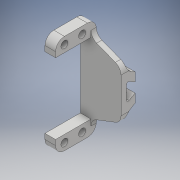
# Autodesk Inventor part: bigServoHolder2
Saved by Autodesk Inventor 2017 (Build 210142000, 142)
## iProperties
Created: 2017-01-16
Part Number: bigServoHolder2
Material: Generic
Document SubType Name: Modeling
Designer: Andi
Density: 1 g/cm^3
Appearance: Default
Author: Andi
Autodesk Inventor part; units mm, degrees
ref_plane "YZ Plane" through (0, 0, 0) normal (1, 0, 0) x (0, 1, 0)
ref_plane "XZ Plane" through (0, 0, 0) normal (0, 1, 0) x (-1, 0, 0)
ref_plane "XY Plane" through (0, 0, 0) normal (0, 0, 1) x (1, 0, 0)
sketch "Sketch1" plane through (0, 0, 0) normal (1, 0, 0) x (0, 1, 0)
  line L0 (0, 0) -> (0, 40)
  line L1 (0, 40) -> (-20, 40)
  line L2 (-20, 40) -> (-20, 43)
  line L3 (-15, 48) -> (-2, 48)
  line L4 (-2, -8) -> (-15, -8)
  line L5 (-20, -3) -> (-20, 0)
  line L6 (-20, 0) -> (0, 0)
  line L7 (0, 20) -> (3, 20)
  line L8 (3, 20) -> (3, 25.5)
  line L9 (3, 23.7768) -> (3, 20)
  line L10 (3, 20) -> (3, 16.2232)
  line L11 (3, 20) -> (7.9, 20)
  line L12 (7.9, 20) -> (7.9, 22.7)
  line L13 (7.9, 22.7) -> (7.9, 20)
  line L14 (7.9, 20) -> (7.9, 17.3)
  line L15 (7.9, 20) -> (10.6, 20) construction
  line L16 (4.4961, 24.6451) -> (7.9, 22.7)
  line L17 (7.9, 17.3) -> (4.4961, 15.3549)
  line L18 (7.9, 17.3) -> (7.9, 12.3)
  line L19 (7.9, 12.3) -> (5.5193, 10.9396)
  line L20 (7.9, 22.7) -> (7.9, 27.7)
  line L21 (7.9, 27.7) -> (5.5193, 29.0604)
  line L22 (3, 43) -> (3, 33.4016)
  line L23 (3, 30.5) -> (3, 25.5)
  line L24 (3, 14.5) -> (3, 9.5)
  line L25 (3, 6.5984) -> (3, -3)
  arc A0 (3, 33.4016) -> (5.5193, 29.0604) centre (8, 33.4016) ccw
  arc A1 (5.5193, 10.9396) -> (3, 6.5984) centre (8, 6.5984) ccw
  arc A2 (-2, -8) -> (3, -3) centre (-2, -3) ccw
  arc A3 (3, 43) -> (-2, 48) centre (-2, 43) ccw
  arc A4 (-15, 48) -> (-20, 43) centre (-15, 43) ccw
  arc A5 (-20, -3) -> (-15, -8) centre (-15, -3) ccw
  arc A6 (3, 16.2232) -> (4.4961, 15.3549) centre (4, 16.2232) ccw
  arc A7 (4.4961, 24.6451) -> (3, 23.7768) centre (4, 23.7768) ccw
  point P0 (-20, 48)
  point P1 (3, 48)
  point P2 (3, -8)
  point P3 (-20, -8)
  point P4 (-20, -1.5)
  dimension "d0" = 40
  dimension "d1" = 20
  dimension "d2" = 8
  dimension "d3" = 23
  dimension "d5" = 56
  dimension "d6" = 23
  dimension "d7" = 5.5
  dimension "d8" = 5.5
  dimension "d9" = 4.9
  dimension "d10" = 2.7
  dimension "d11" = 2.7
  dimension "d13" = 5
  dimension "d14" = 5
  dimension "d15" = 17.5
  dimension "d16" = 17.5
  dimension "d17" = 5
  dimension "d18" = 5
  dimension "d19" = 5
  dimension "d20" = 5
  dimension "d45" = 1
  constraints: 52 end point, 17 point on line, 16 point on circle, 16 tangent, 8 centre point, 5 perpendicular, 5 vertical, 4 collinear, 4 horizontal, 3 equal radius, 3 parallel, 2 midpoint
  measures "d0" distance of L0.start L0.end
  measures "d1" distance of L0.end L1.end
  measures "d2" distance of L1.end point (-20, 48)
  measures "d3" distance of point (-20, 48) point (3, 48)
  measures "d5" distance of point (3, 48) point (3, -8)
  measures "d6" distance of point (3, -8) point (-20, -8)
  measures "d7" distance of L7.end L8.end
  measures "d8" distance of L7.end L24.start
  measures "d9" distance of L7.end L11.end
  measures "d10" distance of L11.end L12.end
  measures "d11" distance of L11.end L14.end
  measures "d13" distance of L14.end L18.end
  measures "d14" distance of L12.end L20.end
  measures "d15" distance of point (3, 48) L23.start
  measures "d16" distance of L24.end point (3, -8)
  measures "d17" radius of A0
  measures "d18" radius of A1
  measures "d19" radius of A2
  measures "d20" radius of A4
  measures "d45" radius of A6
extrude "Extrusion1" add sketch "Sketch1" along normal blind 23 contours L0 L7 L10 A6 L17 L18 L19 A1 L25 A2 L4 A5 L5 L6 | L0 L1 L2 A4 L3 A3 L22 A0 L21 L20 L16 A7 L8 L7
sketch "Sketch2" plane through (0, 0, 0) normal (0, -1, 0) x (1, 0, 0)
  line L0 (0, 48) -> (23, 48) projected
  line L1 (0, 48) -> (6, 48)
  line L2 (6, 48) -> (6, -8)
  line L3 (0, -8) -> (23, -8) projected
  line L4 (0, 6.5984) -> (23, 6.5984) projected
  line L5 (23, 34.6451) -> (23, 6.5984)
  line L6 (23, 6.5984) -> (6, 0)
  line L7 (0, 0) -> (23, 0) projected
  line L8 (23, 33.4016) -> (23, 43) projected
  line L9 (23, 33.4016) -> (6, 40)
  line L10 (0, 40) -> (23, 40) projected
  line L11 (6, 48) -> (23, 48)
  line L12 (23, 33.4016) -> (23, 29.0604) projected
  line L13 (23, 33.4016) -> (23, 48)
  line L14 (23, 6.5984) -> (23, -8)
  line L15 (23, 40) -> (23, 0) projected
  line L16 (6, -8) -> (23, -8)
  dimension "d23" = 6
  constraints: 18 end point, 6 point on line, 3 collinear, 2 perpendicular, 1 horizontal
  measures "d23" distance of L0.start L1.end
extrude "Extrusion2" cut sketch "Sketch2" along normal blind 23 and the other way blind 11.5 contours L0 L13 L8 L10 L2 | L10 L8 L5 L9 | L7 L14 L3 L2 | L6 L14 L7
fillet "Fillet1" radius 5 4 edges at (23, 1.5, 6.5984) (23, 1.5, 33.4016) (6, 1.5, 40) (6, 1.5, 0)
sketch "Sketch3" plane through (0, 0, 0) normal (-1, 0, 0) x (0, 0, 1)
  line L0 (40, 0) -> (0, 0) projected
  line L1 (40, 0) -> (40, -5)
  line L2 (40, -20) -> (40, 0) projected
  line L3 (40, -5) -> (44, -5)
  line L4 (44, -5) -> (44, -15)
  line L5 (0, 0) -> (0, -5)
  line L6 (0, 0) -> (0, -20) projected
  line L7 (0, -5) -> (-4, -5)
  line L8 (-4, -5) -> (-4, -15)
  dimension "d29" = 5
  dimension "d30" = 4
  dimension "d31" = 10
  dimension "d32" = 5
  dimension "d33" = 4
  dimension "d34" = 10
  constraints: 12 end point, 4 perpendicular, 2 point on line
  measures "d29" distance of L0.start L1.end
  measures "d30" distance of L1.end L3.end
  measures "d31" distance of L3.end L4.end
  measures "d32" distance of L0.end L5.end
  measures "d33" distance of L5.end L7.end
  measures "d34" distance of L7.end L8.end
hole "Hole1" at (0, -15, 44) at (0, -5, 44) at (0, -15, -4) at (0, -5, -4) direction (1, 0, 0) diameter 4 depth 15
sketch "Sketch4" plane through (6, -15, -8) normal (1, 0, 0) x (0, 0, -1)
  line L0 (-0.0094, 15) -> (-56.0094, 15)
  line L1 (-56.0094, 15) -> (-56.0094, -8.2095)
  line L2 (-56.0094, -8.2095) -> (-0.0094, -8.2095)
  line L3 (-0.0094, -8.2095) -> (-0.0094, 15)
  point P0 (-8, 15)
  dimension "d42" = 56
  constraints: 8 end point, 2 parallel, 1 horizontal, 1 perpendicular
  measures "d42" distance of L2.end L1.end
extrude "Extrusion3" cut sketch "Sketch4" along normal blind 23
body "Solid1"
